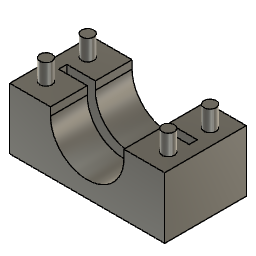
cover (Autodesk Fusion 360 design; units mm, degrees)
Autodesk Fusion 360 part; units mm, degrees
sketch "スケッチ1" plane through (0, 0, 0) normal (0, 0, 1) x (1, 0, 0)
  line L0 (-19, 20) -> (19, 20)
  line L1 (19, 20) -> (19, 0)
  line L2 (19, 0) -> (-19, 0)
  line L3 (-19, 0) -> (-19, 20)
  dimension "d1" = 38
  dimension "d2" = 20
  constraint horizontal L0
  constraint vertical L1
  constraint horizontal L2
  constraint vertical L3
  constraint midpoint origin L2
  measures "d1" distance of L0.start L0.end
  measures "d2" distance of L0.end L1.end
extrude "押し出し1" add sketch "スケッチ1" along normal blind 15
sketch "スケッチ2" plane through (0, 0, 0) normal (0, -1, 0) x (1, 0, 0)
  line L0 (-19, 0) -> (19, 0)
  line L1 (19, 0) -> (19, 15)
  line L2 (19, 15) -> (-19, 15)
  line L3 (-19, 15) -> (-19, 0)
  line L4 (-19, 13) -> (19, 13) construction
  arc A0 (-9, 13) -> (9, 13) centre (0, 13) ccw
  line L5 (9, 13) -> (9, 15)
  line L6 (-9, 13) -> (-9, 15)
  dimension "d5" = 2
  dimension "d6" = 18
  constraint coincident L3 L4.start
  constraint coincident L1 L4.end
  constraint perpendicular L1 L4
  constraint midpoint L4 A0.centre
  constraint coincident L4 A0.end
  constraint coincident L4 A0.start
  constraint coincident L2 L5.end
  constraint tangent A0 L5
  constraint coincident L2 L6.end
  constraint tangent A0 L6
  measures "d5" distance of L2 L4
  measures "d6" diameter of A0
extrude "押し出し2" cut sketch "スケッチ2" against normal blind 20 contours L2 A0 L5 L6
ref_plane "作業平面1" through (0, 9, 7.5) normal (0, -1, 0) x (1, 0, 0)
sketch "スケッチ3" plane through (0, 9, 6.5) normal (0, -1, 0) x (1, 0, 0)
  line L0 (-16, 8.5) -> (16, 8.5)
  line L1 (16, 8.5) -> (16, -4.5)
  line L2 (16, -4.5) -> (-16, -4.5)
  line L3 (-16, -4.5) -> (-16, 8.5)
  line L4 (-19, 8.5) -> (-9, 8.5)
  arc A0 (-9, 6.5) -> (9, 6.5) centre (0, 6.5) ccw
  line L5 (19, -6.5) -> (19, 8.5)
  dimension "d10" = 32
  dimension "d11" = 11
  dimension "d12" = 3
  constraint horizontal L0
  constraint vertical L1
  constraint horizontal L2
  constraint vertical L3
  constraint collinear L0 L4
  measures "d10" distance of L0.start L0.end
  measures "d11" distance of L2 A0.centre
  measures "d12" distance of L1 L5
extrude "押し出し3" cut sketch "スケッチ3" against normal blind 2
sketch "スケッチ4" plane through (0, 0, 15) normal (0, 0, 1) x (-1, 0, 0)
  line L0 (16, -11) -> (9, -11)
  line L1 (9, -11) -> (9, -20)
  line L2 (9, -20) -> (19, -20)
  line L3 (19, -20) -> (19, 0)
  line L4 (19, 0) -> (9, 0)
  line L5 (9, 0) -> (9, -9)
  line L6 (9, -9) -> (16, -9)
  line L7 (16, -9) -> (16, -11)
  line L8 (19, -15.125) -> (-17.5478, -15.125) construction
  line L9 (-19, -20) -> (-9, -20) construction
  line L10 (19, -4.875) -> (-19, -4.875) construction
  line L11 (-19, 0) -> (-19, -20) construction
  circle A0 centre (-15, -15.125) radius 1.5
  circle A1 centre (-15, -4.875) radius 1.5
  circle A2 centre (15, -15.125) radius 1.5
  circle A3 centre (15, -4.875) radius 1.5
  dimension "d15" = 4.875
  dimension "d16" = 10.25
  dimension "d17" = 3
  dimension "d18" = 4
  dimension "d19" = 3
  dimension "d20" = 4
  dimension "d21" = 3
  dimension "d22" = 4
  dimension "d23" = 3
  dimension "d24" = 4
  constraint coincident L3 L8.start
  constraint perpendicular L3 L8
  constraint coincident L3 L10.start
  constraint perpendicular L3 L10
  constraint coincident L10.end L11
  constraint coincident L8 A0.centre
  constraint coincident L10 A1.centre
  constraint coincident L8 A2.centre
  constraint coincident L10 A3.centre
  measures "d15" distance of L8 L9
  measures "d16" distance of L8 L10
  measures "d17" diameter of A0
  measures "d18" distance of L11 A0.centre
  measures "d19" diameter of A1
  measures "d20" distance of L11 A1.centre
  measures "d21" diameter of A2
  measures "d22" distance of L3 A2.centre
  measures "d23" diameter of A3
  measures "d24" distance of L3 A3.centre
extrude "押し出し4" add sketch "スケッチ4" along normal blind 5 contours A0 | A1 | A2 | A3
